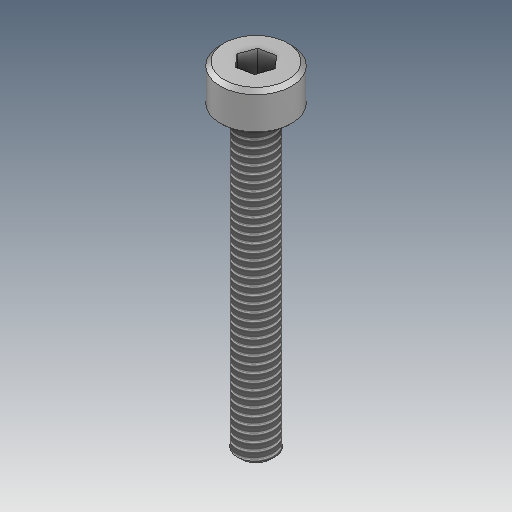
# Autodesk Inventor part: Tornillo Allen cabeza cilindrica M2x16mm
Saved by Autodesk Inventor 2020 (Build 240168000, 168)
## iProperties
Created: 2020-05-08
Part Number: Tornillo Allen cabeza cilindrica M2x16mm
Material: Generic
Document SubType Name: Modeling
Designer: Dante
Density: 1 g/cm^3
Appearance: Goma - Negro - Versión 1.1
Author: Dante
Autodesk Inventor part; units mm, degrees
ref_plane "YZ Plane" through (0, 0, 0) normal (1, 0, 0) x (0, 1, 0)
ref_plane "XZ Plane" through (0, 0, 0) normal (0, 1, 0) x (-1, 0, 0)
ref_plane "XY Plane" through (0, 0, 0) normal (0, 0, 1) x (1, 0, 0)
sketch "Sketch1" plane through (0, 0, 0) normal (0, 0, 1) x (1, 0, 0)
  line L0 (-10.9228, -39) -> (-12.8228, -39)
  line L1 (-12.8228, -39) -> (-12.8228, -37)
  line L2 (-12.8228, -37) -> (-10.9228, -37)
  line L3 (-10.9228, -37) -> (-10.9228, -39)
  line L4 (-10.9228, -39) -> (-10.9228, -55)
  line L5 (-10.9228, -55) -> (-11.9228, -55)
  line L6 (-11.9228, -55) -> (-11.9228, -39)
  point P0 (0, 0)
  dimension "d0" = 1.9
  dimension "d1" = 2
  dimension "d3" = 1
  dimension "d16" = 16
  constraints: 14 end point, 4 perpendicular, 2 vertical, 1 horizontal, 1 point on line
  measures "d0" distance of L0.start L0.end
  measures "d1" distance of L0.end L1.end
  measures "d3" distance of L4.end L5.end
  measures "d16" distance from line of L4.end L0
revolve "Revolution1" add sketch "Sketch1" angle 360 about axis through (-10.9228, -39, 0) along (0, -1, 0)
chamfer "Chamfer1" distance 0.2 angle 45 1 edges at (-9.0228, -37, 0)
sketch "Boceto2" plane through (-10.9228, -37, 0) normal (0, 1, 0) x (1, 0, 0)
  line L0 (0.5669, -0.6547) -> (-0.2835, -0.8183)
  line L1 (-0.2835, -0.8183) -> (-0.8504, -0.1636)
  line L2 (-0.8504, -0.1636) -> (-0.5669, 0.6547)
  line L3 (-0.5669, 0.6547) -> (0.2835, 0.8183)
  line L4 (0.2835, 0.8183) -> (0.8504, 0.1636)
  line L5 (0.8504, 0.1636) -> (0.5669, -0.6547)
  point P0 (10.9228, 0)
  point P1 (0, 0)
  dimension "d11" = 1.5
  constraints: 12 end point, 13 other
  measures "d11" distance between parallel lines of L5 L2
extrude "Extrusión1" cut sketch "Boceto2" against normal blind 2
fillet "Fillet1" radius 0.1 1 edges at (-9.9228, -39, 0)
chamfer "Chamfer3" distance 0.2 angle 45 1 edges at (-9.9228, -55, 0)
thread "Thread2" size "M2x0.4" class "6g" standard "ISO Metric profile" length 98
chamfer "Chamfer4" distance 0.08 angle 45 1 edges at (-9.0228, -39, 0)
body "Solid1"
